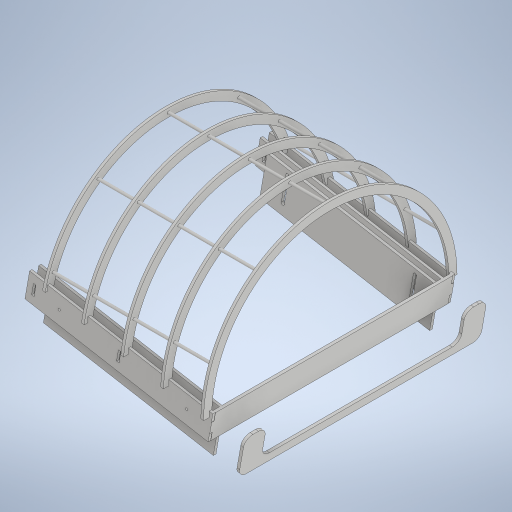
# Autodesk Inventor part: 2020FlatDesign
Saved by Autodesk Inventor 2023 (Build 270158000, 158)
## iProperties
Created: 2021-01-15
Part Number: 2020FlatDesign
Material: Generic
Document SubType Name: Modeling
Designer: Ed
Density: 1 g/cm^3
Appearance: Default
Author: Ed
Autodesk Inventor part; units mm, degrees
note: some values were not read from the file. Chosen so that the rebuilt part matches the saved one: sketch regions of "Extrusion10".
ref_plane "YZ Plane" through (0, 0, 0) normal (1, 0, 0) x (0, 1, 0)
ref_plane "XY Plane" through (0, 0, 0) normal (0, 0, 1) x (1, 0, 0)
sketch "Sketch1" plane through (0, 0, 0) normal (1, 0, 0) x (0, 1, 0)
  arc A0 (0, -279.4) -> (0, 279.4) centre (0, 0) ccw
  arc A1 (0, -298.45) -> (0, 298.45) centre (0, 0) ccw
  line L0 (0, 298.45) -> (0, 279.4)
  line L1 (0, -279.4) -> (0, -298.45)
  arc A2 (0, 298.45) -> (0, -298.45) centre (0, 0) ccw construction
  arc A3 (0, 279.4) -> (0, -279.4) centre (0, 0) ccw construction
  dimension "d0" = 558.8
  dimension "d1" = 596.9
  constraints: 8 point on circle, 4 centre point, 4 end point, 2 coincident, 2 point on line, 1 vertical
  measures "d0" diameter of A0
  measures "d1" diameter of A1
extrude "Extrusion1" add sketch "Sketch1" against normal blind 6.35
pattern_linear "Rectangular Pattern1" count 5 spacing 95.25 along (-1, 0, 0) of "Extrusion1"
ref_plane "Work Plane1" through (0, 0, -298.45) normal (0.1736482, 0.9848078, 0) x (0, 0, 1)
split "Split1" plane through (0, 0, -298.45) removes the side toward (-0.1736482, -0.9848078, 0)
sketch "Sketch2" plane through (0, 0, 0) normal (1, 0, 0) x (0, 0, -1)
  circle A0 centre (0, 288.925) radius 3.175
  line L0 (0, -59.69) -> (0, 358.14) projected
  circle A1 centre (165.7206, 236.6735) radius 3.175
  circle A2 centre (271.5007, 98.8182) radius 3.175
  circle A3 centre (-165.7206, 236.6735) radius 3.175
  circle A4 centre (-271.5007, 98.8182) radius 3.175
  point P0 (0, 0)
  dimension "d9" = 6.35
  dimension "d10" = 288.925
  dimension "d15" = 70
  dimension "d19" = 70
  constraints: 5 centre point, 1 point on line, 10 other
  measures "d9" diameter of A0
  measures "d10" distance of point (0, 0) A0.centre
extrude "Extrusion2" cut sketch "Sketch2" against normal through all
ref_plane "Work Plane3" through (0, 0, 279.4) normal (-0.9848078, 0.1736482, 0) x (0, 0, 1)
sketch "Sketch4" plane through (0, 0, 279.4) normal (-0.9848078, 0.1736482, 0) x (0, 0, 1)
  line L0 (-697.23, 0) -> (138.43, 0) projected
  ellipse E0 centre (-279.4, 0) end of major axis (-558.8, 0) minor radius 275.1553 (-0.2978, 0) -> (-558.8, 0) ccw projected
  line L1 (-279.4, -141.2709) -> (-279.4, 376.7868) projected
  line L2 (-577.85, 0) -> (-558.8, 0) projected
  line L3 (5.842, 12.7) -> (0, 12.7)
  line L4 (0, 12.7) -> (0, 0)
  line L5 (0, 0) -> (5.842, 0)
  line L6 (5.842, 0) -> (5.842, 12.7)
  line L7 (5.842, 0) -> (0, 0)
  line L8 (0, 0) -> (0, -50.8)
  line L9 (0, -50.8) -> (5.842, -50.8)
  line L10 (5.842, -50.8) -> (5.842, 0)
  line L11 (-558.8, 12.7) -> (-564.642, 12.7)
  line L12 (-564.642, 12.7) -> (-564.642, 0)
  line L13 (-564.642, 0) -> (-558.8, 0)
  line L14 (-558.8, 0) -> (-558.8, 12.7)
  line L15 (-564.642, 0) -> (-558.8, 0)
  line L16 (-558.8, 0) -> (-558.8, -50.8)
  line L17 (-558.8, -50.8) -> (-564.642, -50.8)
  line L18 (-564.642, -50.8) -> (-564.642, 0)
  dimension "d48" = 5.842
  dimension "d49" = 12.7
  dimension "d50" = 5.842
  dimension "d51" = 50.8
  dimension "d52" = 5.842
  dimension "d53" = 12.7
  dimension "d54" = 50.8
  dimension "d55" = 5.842
  constraints: 32 end point, 8 parallel, 4 horizontal, 4 perpendicular, 2 collinear, 3 other
  measures "d48" distance of L3.start L3.end
  measures "d49" distance of L5.end L3.start
  measures "d50" distance of L8.end L9.end
  measures "d51" distance of L7.end L8.end
  measures "d52" distance of L11.start L11.end
  measures "d53" distance of L11.end L12.end
  measures "d54" distance of L17.end L12.end
  measures "d55" distance of L16.end L17.end
extrude "Extrusion4" add sketch "Sketch4" along normal blind 431.8 contours L12 L11 L14 L0 | L4 L3 L6 L0 | L0 L10 L9 L8 | L0 L16 L17 L18
extrude "Extrusion6" add sketch "Sketch4" against normal blind 6.35 contours L12 L11 L14 L0 | L4 L3 L6 L0 | L0 L10 L9 L8 | L0 L16 L17 L18
sketch "Sketch7" plane through (0, 0, 285.242) normal (0, 0, 1) x (1, 0, 0)
  line L0 (5.1509, -7.3562) -> (0.7402, -32.3703)
  line L1 (0.7402, -32.3703) -> (-5.013, -31.3559)
  line L2 (-5.013, -31.3559) -> (-0.6024, -6.3417)
  line L3 (-0.6024, -6.3417) -> (5.1509, -7.3562)
  line L4 (8.4589, 11.4044) -> (-2.5678, -51.1309) projected
  point P0 (0, 0)
  point P1 (2.9455, -19.8633)
  dimension "d58" = 5.842
  dimension "d59" = 25.4
  constraints: 8 end point, 2 midpoint, 2 parallel, 1 collinear, 1 perpendicular
  measures "d58" distance of L0.end L1.end
  measures "d59" distance of L1.end L2.end
extrude "Extrusion7" cut sketch "Sketch7" against normal through all
sketch "Sketch6" plane through (0, 0, 279.4) normal (-0.9848078, 0.1736482, 0) x (0, 0, 1)
  circle A0 centre (-279.4, 0) radius 304.8
  line L0 (-845.8416, 0) -> (304.3447, 0) projected
  line L1 (-279.4, -665.4254) -> (-279.4, 560.5152) projected
  line L2 (-21.479, -72.9288) -> (-537.321, -72.9288)
  point P0 (-279.4, -72.9288)
  dimension "d42" = 0
  dimension "d43" = 0
  dimension "d44" = 609.6
  dimension "d45" = 515.842
  constraints: 2 end point, 1 centre point, 1 horizontal, 1 midpoint, 1 point on line
  measures "d42" distance from line of L0 A0.centre
  measures "d43" distance from line of L1 A0.centre
  measures "d44" diameter of A0
  measures "d45" distance of L2.start L2.end
sketch "Sketch8" plane through (-0.6024, -6.3417, 285.242) normal (0.9848078, -0.1736482, 0) x (0, 0, -1)
  line L0 (5.842, 0) -> (5.842, 19.05) projected
  line L1 (5.842, 19.05) -> (5.842, 0)
  line L2 (5.842, 0) -> (0, 0)
  line L3 (0, 0) -> (0, -25.4)
  line L4 (5.842, -25.4) -> (0, -25.4) projected
  line L5 (0, -25.4) -> (5.842, -25.4)
  line L6 (0, -44.45) -> (5.842, -44.45) projected
  line L7 (5.842, -25.4) -> (5.842, -44.45)
  line L8 (5.842, -44.45) -> (564.642, -44.45)
  line L9 (564.642, -44.45) -> (564.642, -25.4)
  line L10 (564.642, -44.45) -> (564.642, 19.05) projected
  line L11 (564.642, -25.4) -> (570.484, -25.4) projected
  line L12 (570.484, -25.4) -> (570.484, 0)
  line L13 (570.484, 19.05) -> (570.484, -44.45) projected
  line L14 (564.642, 0) -> (570.484, 0) projected
  line L15 (570.484, 19.05) -> (564.642, 19.05) projected
  line L16 (564.642, 0) -> (564.642, 19.05)
  line L17 (564.642, 19.05) -> (5.842, 19.05)
  point P0 (285.242, 6.35)
  constraints: 20 end point, 6 perpendicular, 4 point on line, 2 collinear
extrude "Extrusion8" add sketch "Sketch8" along normal blind 6.35 contours L0 L17 L10 L9 L8 L7 L4 L3 L2 | L14 L12 L11 L10
ref_plane "Work Plane4" through (-12.664, -71.8209, 257.921) normal (0, 0, 1) x (1, 0, 0)
sketch "Sketch10" plane through (-12.664, -71.8209, 257.921) normal (0, 0, 1) x (1, 0, 0)
  line L0 (4.3429, 21.7044) -> (15.3696, 84.2397) projected
  line L1 (15.3696, 84.2397) -> (4.3429, 21.7044) projected
  line L2 (-421.3974, 96.7739) -> (4.3429, 21.7044)
  line L3 (4.3429, 21.7044) -> (15.3696, 84.2397)
  line L4 (15.3696, 84.2397) -> (-410.3707, 159.3092)
  line L5 (-410.3707, 159.3092) -> (-421.3974, 96.7739)
  line L6 (7.6509, 40.465) -> (12.0616, 65.4791)
  line L7 (12.0616, 65.4791) -> (17.8148, 64.4647)
  line L8 (17.8148, 64.4647) -> (13.4042, 39.4506)
  line L9 (13.4042, 39.4506) -> (7.6509, 40.465)
  line L10 (-405.5823, 113.3292) -> (-401.1716, 138.3433)
  line L11 (-401.1716, 138.3433) -> (-395.4184, 137.3289)
  line L12 (-395.4184, 137.3289) -> (-399.8291, 112.3147)
  line L13 (-399.8291, 112.3147) -> (-405.5823, 113.3292)
  line L14 (-415.884, 128.0416) -> (15.6095, 51.9576)
  line L15 (-205.4694, 78.0439) -> (-201.0587, 103.058)
  line L16 (-201.0587, 103.058) -> (-195.3055, 102.0435)
  line L17 (-195.3055, 102.0435) -> (-199.7161, 77.0294)
  line L18 (-199.7161, 77.0294) -> (-205.4694, 78.0439)
  line L19 (-421.3974, 96.7739) -> (4.3429, 21.7044)
  circle A0 centre (-40.6723, 61.8816) radius 2.54
  circle A1 centre (-340.8417, 114.8096) radius 2.54
  point P0 (12.664, 71.8209)
  point P1 (9.8562, 52.9721)
  point P2 (-403.377, 125.8363)
  point P3 (-203.264, 90.5509)
  dimension "d67" = 5.842
  dimension "d68" = 25.4
  dimension "d69" = 5.842
  dimension "d70" = 25.4
  dimension "d71" = 62.5353
  dimension "d72" = 12.7
  dimension "d75" = 5.842
  dimension "d76" = 25.4
  dimension "d77" = 215.9
  dimension "d83" = 5.08
  dimension "d84" = 5.08
  dimension "d85" = 76.2
  dimension "d86" = 381
  constraints: 36 end point, 9 parallel, 6 midpoint, 5 perpendicular, 4 point on line, 2 centre point
  measures "d67" distance of L6.end L7.end
  measures "d68" distance of L7.end L8.end
  measures "d69" distance of L10.end L11.end
  measures "d70" distance of L11.end L12.end
  measures "d71" vertical distance of L4.end L2.start
  measures "d72" distance between parallel lines of L5 L10
  measures "d75" distance of L15.end L16.end
  measures "d76" distance of L15.start L15.end
  measures "d77" distance between parallel lines of L15 L5
  measures "d83" diameter of A0
  measures "d84" diameter of A1
  measures "d85" distance from line of A1.centre L5
  measures "d86" distance from line of A0.centre L5
extrude "Extrusion10" add sketch "Sketch10" along normal blind 5.842 contours L2 L5 L14 L10 L13 L12 A1 L15 L18 L17 A0 L0 | L0 L14 L8 L9 | L14 A0 L17 L16 L15 A1 L12 L11 L10 L5 L4 L0 | L0 L7 L8 L14 | A0 L14 | L14 A0 | A1 L14 | L14 A1
mirror "Mirror1" about plane through (0, 0, 0) normal (0, 0, 1) of "Extrusion10"
extrude "Extrusion11" cut sketch "Sketch10" along normal through all both and the other way through all contours A0 L14 | L14 A0 | L14 L12 L13 L10 | L10 L11 L12 L14 | L17 L18 L15 L14 | L14 L15 L16 L17 | A1 L14 | L14 A1
sketch "Sketch11" plane through (-387.35, 0, 0) normal (-1, 0, 0) x (0, 0, 1)
  arc A0 (278.8251, 17.9148) -> (-278.8251, 17.9148) centre (0, 0) ccw projected
  line L0 (279.4, 67.1806) -> (271.2031, 67.1806) projected
  line L1 (0, 0) -> (271.2031, 67.1806)
  line L2 (-279.4, 68.3003) -> (-270.9233, 68.3003) projected
  line L3 (-270.9233, 68.3003) -> (0, 0)
  dimension "d87" = 151.938
  constraints: 4 end point
  measures "d87" angle of L1 L3
sketch "Sketch12" plane through (0, 0, 257.921) normal (0, 0, 1) x (1, 0, 0)
  line L0 (-400.2259, 70.5706) -> (0, 0)
  line L1 (0, 0) -> (-17.6427, -100.0565)
  line L2 (-17.6427, -100.0565) -> (-417.8685, -29.4858)
  line L3 (-417.8685, -29.4858) -> (-400.2259, 70.5706)
  line L4 (-434.0613, 24.953) -> (-2.5678, -51.1309) projected
  line L5 (-434.0613, 24.953) -> (-423.0347, 87.4883) projected
  line L6 (-52.2336, -3.6857) -> (-63.2602, -66.221) construction
  line L7 (-55.7355, -3.0682) -> (-66.7622, -65.6035)
  line L8 (-59.7582, -66.8385) -> (-48.7316, -4.3032)
  arc A0 (-48.7316, -4.3032) -> (-55.7355, -3.0682) centre (-52.2336, -3.6857) ccw
  arc A1 (-66.7622, -65.6035) -> (-59.7582, -66.8385) centre (-63.2602, -66.221) ccw
  line L9 (-200.1129, 35.2853) -> (-217.7556, -64.7712) construction
  line L10 (-352.403, 49.2422) -> (-363.4296, -13.2931) construction
  line L11 (-348.901, 48.6247) -> (-359.9277, -13.9106)
  line L12 (-366.9316, -12.6756) -> (-355.9049, 49.8597)
  arc A2 (-348.901, 48.6247) -> (-355.9049, 49.8597) centre (-352.403, 49.2422) ccw
  arc A3 (-366.9316, -12.6756) -> (-359.9277, -13.9106) centre (-363.4296, -13.2931) ccw
  line L13 (-292.1, 64.401) -> (-381, 80.0765) projected
  point P0 (0, 0)
  point P1 (-57.7469, -34.9534)
  point P2 (-357.9163, 17.9746)
  point P3 (-353.5056, 42.9887)
  point P4 (-357.9163, 17.9746)
  dimension "d88" = 406.4
  dimension "d89" = 101.6
  dimension "d90" = 31.75
  dimension "d91" = 7.112
  dimension "d92" = 152.4
  dimension "d93" = 12.7
  dimension "d96" = 44.45
  constraints: 26 end point, 8 point on circle, 7 symmetric about line, 4 centre point, 4 midpoint, 4 parallel, 4 tangent, 2 perpendicular, 1 point on line, 2 other
  measures "d88" distance of L0.start L0.end
  measures "d89" distance of L0.end L1.end
  measures "d90" distance of point (-57.747, -34.953) L6.end
  measures "d91" diameter of A1
  measures "d92" distance between parallel lines of L9 L6
  measures "d93" distance between parallel lines of L0 L13
  measures "d96" distance from line of L0 point (-357.916, 17.975)
extrude "Extrusion12" add sketch "Sketch12" against normal blind 6.35 contours L0 L1 L4 L8 A0 L7 L11 A2 L12 L3 | L4 L12 A3 L11 L7 A1 L8 L1 L2 L3
mirror "Mirror2" about plane through (0, 0, 0) normal (0, 0, 1) of "Extrusion12"
ref_plane "Work Plane6" through (80.6935, -20.6764, 285.242) normal (0.9848078, -0.1736482, 0) x (0, 0, -1)
sketch "Sketch14" plane through (80.6935, -20.6764, 285.242) normal (0.9848078, -0.1736482, 0) x (0, 0, -1)
  arc A0 (50.8001, -0.3432) -> (31.7133, 18.7435) centre (31.7133, -0.3432) ccw
  line L0 (31.7133, 18.7435) -> (19.0868, 18.7435)
  arc A1 (19.0868, 18.7435) -> (0, -0.3432) centre (19.0868, -0.3432) ccw
  line L1 (0, -0.3432) -> (0, -51.0698)
  arc A2 (0, -51.0698) -> (19.0868, -70.1565) centre (19.0868, -51.0698) ccw
  line L2 (19.0868, -70.1565) -> (551.3942, -70.1565)
  arc A3 (551.3942, -70.1565) -> (570.481, -51.0698) centre (551.3942, -51.0698) ccw
  line L3 (570.481, -51.0698) -> (570.481, -0.3432)
  arc A4 (570.481, -0.3432) -> (551.3942, 18.7435) centre (551.3942, -0.3432) ccw
  line L4 (551.3942, 18.7435) -> (538.7708, 18.7435)
  arc A5 (538.7708, 18.7435) -> (519.6841, -0.3432) centre (538.7708, -0.3432) ccw
  line L5 (519.6841, -0.3432) -> (519.6841, -31.983)
  arc A6 (500.5973, -51.0698) -> (519.6841, -31.983) centre (500.5973, -31.983) ccw
  line L6 (500.5973, -51.0698) -> (69.8869, -51.0698)
  arc A7 (50.8001, -31.983) -> (69.8869, -51.0698) centre (69.8869, -31.983) ccw
  line L7 (50.8001, -31.983) -> (50.8001, -0.3432)
  point P0 (285.242, 6.35)
  dimension "d1" = 596.9
  dimension "d106" = 532.3075
  dimension "d107" = 12.6265
  dimension "d108" = 12.6234
  dimension "d109" = 50.7265
  dimension "d110" = 38.1736
  dimension "d111" = 38.1736
  dimension "d112" = 38.1736
  constraints: 17 tangent, 16 end point, 16 point on circle, 8 centre point, 7 equal radius, 4 perpendicular, 2 parallel, 1 collinear
  measures "d106" distance of A3.centre A2.centre
  measures "d107" distance of A0.centre A1.centre
  measures "d108" distance of A4.centre A5.centre
  measures "d109" distance of A3.centre A4.centre
  measures "d110" horizontal distance of A7.centre A0.centre
  measures "d111" horizontal distance of A6.centre A5.centre
  measures "d112" distance from line of L2 A6.centre
extrude "Extrusion14" add sketch "Sketch14" against normal blind 6.35
sketch "Sketch15" plane through (0, 0, 0) normal (1, 0, 0) x (0, 0, -1)
  circle A0 centre (-271.5007, 98.8182) radius 3.175 projected
  circle A1 centre (-165.7206, 236.6735) radius 3.175 projected
  circle A2 centre (0, 288.925) radius 3.175 projected
  circle A3 centre (165.7206, 236.6735) radius 3.175 projected
  circle A4 centre (271.5007, 98.8182) radius 3.175 projected
  point P0 (0, 0)
extrude "Extrusion15" add sketch "Sketch15" against normal up to surface (387.35 mm away)
sketch "Sketch13" plane through (80.6935, -20.6764, 285.242) normal (0.9848078, -0.1736482, 0) x (0, 0, -1)
  line L0 (31.7133, 654.05) -> (19.0868, 654.05)
  line L1 (50.8001, 622.3367) -> (50.8001, 634.9632)
  arc A0 (50.8001, 634.9632) -> (31.7133, 654.05) centre (31.7133, 634.9632) ccw
  line L2 (500.5973, 603.2499) -> (69.8869, 603.2499)
  arc A1 (50.8001, 622.3367) -> (69.8869, 603.2499) centre (69.8869, 622.3367) ccw
  line L3 (519.6841, 634.9632) -> (519.6841, 622.3367)
  arc A2 (500.5973, 603.2499) -> (519.6841, 622.3367) centre (500.5973, 622.3367) ccw
  line L4 (551.3942, 654.05) -> (538.7708, 654.05)
  arc A3 (538.7708, 654.05) -> (519.6841, 634.9632) centre (538.7708, 634.9632) ccw
  line L5 (570.481, 584.2367) -> (570.481, 634.9632)
  arc A4 (570.481, 634.9632) -> (551.3942, 654.05) centre (551.3942, 634.9632) ccw
  line L6 (19.0868, 565.1499) -> (551.3942, 565.1499)
  arc A5 (551.3942, 565.1499) -> (570.481, 584.2367) centre (551.3942, 584.2367) ccw
  line L7 (0, 634.9632) -> (0, 584.2367)
  arc A6 (0, 584.2367) -> (19.0868, 565.1499) centre (19.0868, 584.2367) ccw
  arc A7 (19.0868, 654.05) -> (0, 634.9632) centre (19.0868, 634.9632) ccw
  line L8 (0, 0) -> (0, -25.4) projected
  point P0 (285.242, 6.35)
  point P1 (570.481, 609.6)
  point P2 (0, 609.6)
  point P3 (519.6841, 628.65)
  point P4 (50.8001, 628.65)
  dimension "d1" = 596.9
  dimension "d98" = 570.481
  dimension "d99" = 38.1
  dimension "d100" = 50.797
  dimension "d101" = 88.9001
  dimension "d102" = 468.884
  constraints: 17 tangent, 16 end point, 16 point on circle, 8 centre point, 7 equal radius, 4 midpoint, 4 perpendicular, 2 collinear, 2 parallel
  measures "d98" distance of point (570.481, 609.6) point (0, 609.6)
  measures "d99" distance between parallel lines of L6 L2
  measures "d100" distance from line of L5 point (519.684, 628.65)
  measures "d101" distance from line of L6 L4.end
  measures "d102" distance of point (519.684, 628.65) point (50.8, 628.65)
sketch "Sketch9" plane through (-12.664, -71.8209, 257.921) normal (0, 0, 1) x (1, 0, 0)
  line L0 (-410.3707, 159.3092) -> (15.3696, 84.2397)
  line L1 (15.3696, 84.2397) -> (-6.6837, -40.8308)
  line L2 (-6.6837, -40.8308) -> (-432.424, 34.2386)
  line L3 (-432.424, 34.2386) -> (-410.3707, 159.3092)
  line L4 (-421.3974, 96.7739) -> (10.0962, 20.69) projected
  line L5 (-421.3974, 96.7739) -> (-410.3707, 159.3092) projected
  line L6 (15.3696, 84.2397) -> (4.3429, 21.7044) projected
  line L7 (-374.686, 153.0171) -> (-410.3707, 159.3092) projected
  point P0 (12.664, 71.8209)
  dimension "d64" = 127
  constraints: 8 end point, 3 collinear, 3 parallel, 1 perpendicular
  measures "d64" distance of L0.end L1.end
ref_plane "Work Plane5" through (0, 0, 0) normal (0, 0, 1) x (1, 0, 0)
equation "\"d112\" = d110"
body "Solid1"
